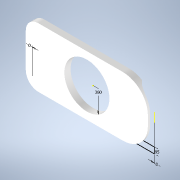
# Autodesk Inventor part: XPS
Saved by Autodesk Inventor 2020.3 (Build 243373010, 373A)
## iProperties
Created: 2021-02-04
Part Number: XPS
Material: Polystyrol
Document SubType Name: Modeling
Designer: Stefan
Density: 1.021 g/cm^3
Appearance: Glatt - Weiß
Author: Stefan
Autodesk Inventor part; units mm, degrees
ref_plane "YZ Plane" through (0, 0, 0) normal (1, 0, 0) x (0, 1, 0)
ref_plane "XZ Plane" through (0, 0, 0) normal (0, 1, 0) x (-1, 0, 0)
ref_plane "XY Plane" through (0, 0, 0) normal (0, 0, 1) x (1, 0, 0)
sketch "Skizze2" plane through (0, 0, 0) normal (0, 0, 1) x (1, 0, 0)
  line L0 (-775, 525) -> (575, 525)
  line L1 (975, 125) -> (975, -25)
  line L2 (575, -425) -> (-775, -425)
  line L3 (-975, -225) -> (-975, 325)
  arc A0 (975, 125) -> (575, 525) centre (575, 125) ccw
  arc A1 (575, -425) -> (975, -25) centre (575, -25) ccw
  arc A2 (-775, 525) -> (-975, 325) centre (-775, 325) ccw
  arc A3 (-975, -225) -> (-775, -425) centre (-775, -225) ccw
  circle A4 centre (0, 50) radius 360
  point P0 (0, 0)
  point P1 (975, -425)
  point P2 (975, 525)
  point P3 (-975, -425)
  dimension "d0" = 950
  dimension "d1" = 1950
  dimension "d2" = 400
  dimension "d3" = 200
  dimension "d4" = 720
  dimension "d5" = 975
  dimension "d6" = 475
  constraints: 8 end point, 8 point on circle, 8 tangent, 6 point on line, 5 centre point, 2 equal radius, 2 parallel, 1 coincident, 1 horizontal, 1 perpendicular
  measures "d0" distance of point (975, 525) point (975, -425)
  measures "d1" distance of point (975, -425) point (-975, -425)
  measures "d2" radius of A0
  measures "d3" radius of A2
  measures "d4" diameter of A4
  measures "d5" distance from line of L1 A4.centre
  measures "d6" distance from line of L0 A4.centre
extrude "Extrusion1" add sketch "Skizze2" against normal blind 100
sketch "Skizze3" plane through (-775, -425, 0) normal (0, -1, 0) x (1, 0, 0)
  line L0 (1750, 0) -> (1350, 0) projected
  line L1 (1350, -100) -> (1750, -100) projected
  line L2 (1350, 0) -> (1750, 0)
  line L3 (1750, 0) -> (1750, -100)
  line L4 (1750, -100) -> (1350, -100)
  line L5 (1350, -100) -> (1350, 0)
  line L6 (1750, -100) -> (1679.3683, -100)
  line L7 (1670, -35) -> (1750, -35)
  line L8 (1750, -35) -> (1750, -100)
  ellipse E0 centre (1679.3683, -100) end of major axis (1670, -35) minor radius 127.378 (1670, -35) -> (1555.4261, -100) ccw
  point P0 (775, 0)
  dimension "d11" = 65
  dimension "d12" = 80
  constraints: 14 end point, 3 parallel, 2 horizontal, 1 perpendicular, 1 point on line, 4 other
  measures "d11" distance between parallel lines of L1 L7
  measures "d12" distance of L7.start L7.end
extrude "Extrusion2" cut sketch "Skizze3" against normal through all contours L3 L1 E0 L7
sketch "Skizze4" plane through (0, 0, -100) normal (0, 0, -1) x (-1, 0, 0)
  line L0 (975, -410) -> (-975, -410)
  line L1 (-975, -410) -> (-975, -315)
  line L2 (-975, -315) -> (975, -315)
  line L3 (975, -315) -> (975, -410)
  line L4 (975, -225) -> (975, 325) projected
  line L5 (-975, -25) -> (-975, 125) projected
  line L6 (-575, -425) -> (775, -425) projected
  line L7 (975, 415) -> (-975, 415)
  line L8 (-975, 415) -> (-975, 510)
  line L9 (-975, 510) -> (975, 510)
  line L10 (975, 510) -> (975, 415)
  line L11 (775, 525) -> (-575, 525) projected
  point P0 (0, 0)
  dimension "d15" = 95
  dimension "d16" = 0
  dimension "d17" = 0
  dimension "d19" = 15
  dimension "d20" = 95
  dimension "d21" = 0
  dimension "d22" = 0
  dimension "d23" = 15
  constraints: 16 end point, 4 parallel, 2 horizontal, 2 perpendicular
  measures "d15" distance of L0.end L1.end
  measures "d16" distance between parallel lines of L4 L3
  measures "d17" distance between parallel lines of L5 L1
  measures "d19" distance between parallel lines of L6 L0
  measures "d20" distance of L7.end L8.end
  measures "d21" distance between parallel lines of L4 L10
  measures "d22" distance between parallel lines of L5 L8
  measures "d23" distance between parallel lines of L11 L9
extrude "Extrusion3" cut sketch "Skizze4" against normal blind 20
